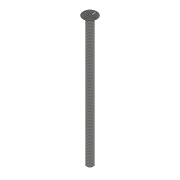
# Autodesk Inventor part: m2_40mm
Saved by Autodesk Inventor 2021 (Build 250183000, 183)
## iProperties
Created: 2022-10-18
Part Number: m2_40mm
Material: Stainless Steel
Document SubType Name: Modeling
Designer: alyn649
Density: 8 g/cm^3
Appearance: Steel - Polished
Author: alyn649
Autodesk Inventor part; units mm, degrees
ref_plane "YZ Plane" through (0, 0, 0) normal (1, 0, 0) x (0, 1, 0)
ref_plane "XZ Plane" through (0, 0, 0) normal (0, 1, 0) x (-1, 0, 0)
sketch "Sketch1" plane through (0, 0, 0) normal (0, 1, 0) x (-1, 0, 0)
  circle A0 centre (0, 0) radius 1
  dimension "d0" = 2
  constraints: 1 centre point, 1 coincident
  measures "d0" diameter of A0
extrude "Extrusion1" add sketch "Sketch1" along normal blind 40
sketch "Sketch2" plane through (0, 40, 0) normal (0, 1, 0) x (1, 0, 0)
  circle A0 centre (0, 0) radius 2.1
  dimension "d3" = 4.2
  constraints: 1 centre point, 1 coincident
  measures "d3" diameter of A0
ref_plane "Work Plane1" through (0, 39, 0) normal (0, 1, 0) x (1, 0, 0)
sketch "Sketch3" plane through (0, 39, 0) normal (0, 1, 0) x (1, 0, 0)
  circle A0 centre (0, 0) radius 1 projected
loft "Loft1" add profiles "Sketch3", "Sketch2"
sketch "Sketch4" plane through (0, 40, 0) normal (0, 1, 0) x (1, 0, 0)
  line L0 (-1.7, -0.3) -> (1.7, -0.3)
  line L1 (1.7, -0.3) -> (1.7, 0.3)
  line L2 (1.7, 0.3) -> (-1.7, 0.3)
  line L3 (-1.7, 0.3) -> (-1.7, -0.3)
  line L4 (-0.3, -1.7) -> (0.3, -1.7)
  line L5 (0.3, -1.7) -> (0.3, 1.7)
  line L6 (0.3, 1.7) -> (-0.3, 1.7)
  line L7 (-0.3, 1.7) -> (-0.3, -1.7)
  point P0 (0, 0)
  point P1 (-1.7, 0)
  point P2 (0, -1.7)
  point P3 (0, -0.3)
  point P4 (0.3, 0)
  point P5 (-0.3, -0.3)
  point P6 (0.3, -0.3)
  point P7 (0.3, 0.3)
  point P8 (-0.3, 0.3)
  dimension "d9" = 3.4
  dimension "d10" = 3.4
  dimension "d11" = 0.6
  dimension "d12" = 0.6
  constraints: 16 end point, 4 midpoint, 4 parallel, 2 horizontal, 2 horizontal alignment, 2 perpendicular, 2 vertical alignment
  measures "d9" distance of L6.end L4.start
  measures "d10" distance of L1.end L2.end
  measures "d11" distance of L2.end L0.start
  measures "d12" distance of L4.start L4.end
extrude "Extrusion2" cut sketch "Sketch4" against normal blind 0.3
chamfer "Chamfer1" distance 0.3 distance2 1 1 edges at (1.7, 39.7, 0) measured on face at (1.7, 39.9, 0.1)
chamfer "Chamfer2" distance 0.3 distance2 1 1 edges at (0, 39.7, 1.7) measured on face at (-0.1, 39.9, 1.7)
chamfer "Chamfer3" distance 0.3 distance2 1 1 edges at (-1.7, 39.7, 0) measured on face at (-1.7, 39.9, -0.1)
chamfer "Chamfer4" distance 0.3 distance2 1 1 edges at (0, 39.7, -1.7) measured on face at (0.1, 39.9, -1.7)
fillet "Fillet1" radius 0.4 4 edges at (0.3, 39.85, 0.3) (-0.3, 39.85, 0.3) (0.3, 39.85, -0.3) (-0.3, 39.85, -0.3)
thread "Thread1" size "M2x0.4" class "6g" standard "ANSI Metric M Profile" full length
equation "\"d12\" = d11"
body "Solid1"
